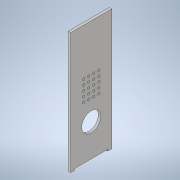
# Autodesk Inventor part: inner_3Poke
Saved by Autodesk Inventor 2020 (Build 240168000, 168)
## iProperties
Created: 2018-12-12
Part Number: inner_3Poke
Material: Generic
Document SubType Name: Modeling
Designer: aonih
Density: 1 g/cm^3
Appearance: Default
Author: aonih
Autodesk Inventor part; units mm, degrees
ref_plane "YZ Plane" through (0, 0, 0) normal (1, 0, 0) x (0, 1, 0)
ref_plane "XZ Plane" through (0, 0, 0) normal (0, 1, 0) x (-1, 0, 0)
ref_plane "XY Plane" through (0, 0, 0) normal (0, 0, 1) x (1, 0, 0)
sketch "Sketch1" plane through (0, 0, 0) normal (1, 0, 0) x (0, 1, 0)
  line L0 (119.0767, 81.9121) -> (-121.9233, 81.9121)
  line L1 (-121.9233, 81.9121) -> (-121.9233, -0.0879)
  line L2 (-121.9233, -0.0879) -> (119.0767, -0.0879)
  line L3 (119.0767, -0.0879) -> (119.0767, 81.9121)
  circle A0 centre (-54.9233, 40.9121) radius 19
  line L4 (-121.9233, 73.9121) -> (-118.9233, 73.9121)
  line L5 (-118.9233, 73.9121) -> (-118.9233, 7.9121)
  line L6 (-118.9233, 7.9121) -> (-121.9233, 7.9121)
  line L7 (-121.9233, 7.9121) -> (-121.9233, 73.9121)
  circle A1 centre (26.2941, 56.2319) radius 2.35
  circle A2 centre (16.2941, 56.2319) radius 2.35
  circle A3 centre (6.2941, 56.2319) radius 2.35
  circle A4 centre (-3.7059, 56.2319) radius 2.35
  circle A5 centre (-13.7059, 56.2319) radius 2.35
  circle A6 centre (26.2941, 46.2319) radius 2.35
  circle A7 centre (16.2941, 46.2319) radius 2.35
  circle A8 centre (6.2941, 46.2319) radius 2.35
  circle A9 centre (-3.7059, 46.2319) radius 2.35
  circle A10 centre (-13.7059, 46.2319) radius 2.35
  circle A11 centre (26.2941, 36.2319) radius 2.35
  circle A12 centre (16.2941, 36.2319) radius 2.35
  circle A13 centre (6.2941, 36.2319) radius 2.35
  circle A14 centre (-3.7059, 36.2319) radius 2.35
  circle A15 centre (-13.7059, 36.2319) radius 2.35
  circle A16 centre (26.2941, 26.2319) radius 2.35
  circle A17 centre (16.2941, 26.2319) radius 2.35
  circle A18 centre (6.2941, 26.2319) radius 2.35
  circle A19 centre (-3.7059, 26.2319) radius 2.35
  circle A20 centre (-13.7059, 26.2319) radius 2.35
  point P0 (0, 0)
  point P1 (0, 0)
  dimension "d0" = 241
  dimension "d1" = 82
  dimension "d2" = 38
  dimension "d3" = 41
  dimension "d4" = 174
  dimension "d5" = 66
  dimension "d6" = 3
  dimension "d7" = 8
  dimension "d21" = 4.7
  dimension "d24" = 10
  dimension "d27" = 10
  constraints: 21 centre point, 16 end point, 4 parallel, 3 horizontal, 2 perpendicular, 1 coincident, 1 point on line, 1 vertical
  measures "d0" distance of L1.end L2.end
  measures "d1" distance of L2.end L0.start
  measures "d2" diameter of A0
  measures "d3" distance from line of L0 A0.centre
  measures "d4" distance from line of L3 A0.centre
  measures "d5" distance of L4.end L5.end
  measures "d6" distance of L5.end L6.end
  measures "d7" distance from line of L2 L5.end
  measures "d21" diameter of A1
  measures "d24" distance of A1.centre A2.centre
  measures "d27" distance of A1.centre A6.centre
extrude "Extrusion1" add sketch "Sketch1" along normal blind 5 contours L3 L2 L1 L6 L5 L4 L0
equation "\"d3\" = 0.5 * d1"
equation "\"d7\" = -0.5 * d5 + 0.5 * d1"
body "Solid1"
